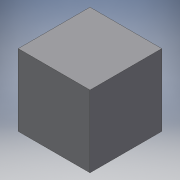
# Autodesk Inventor part: Y screw nut
Saved by Autodesk Inventor 2019 (Build 230136000, 136)
## iProperties
Created: 2018-10-07
Part Number: Y screw nut
Material: Generic
Document SubType Name: Modeling
Designer: LillaHunden
Density: 1 g/cm^3
Appearance: Default
Author: LillaHunden
Autodesk Inventor part; units mm, degrees
ref_plane "YZ Plane" through (0, 0, 0) normal (1, 0, 0) x (0, 1, 0)
ref_plane "XZ Plane" through (0, 0, 0) normal (0, 1, 0) x (-1, 0, 0)
ref_plane "XY Plane" through (0, 0, 0) normal (0, 0, 1) x (1, 0, 0)
sketch "Sketch1" plane through (0, 0, 0) normal (0, 0, 1) x (1, 0, 0)
  line L0 (11, -11) -> (-11, -11)
  line L1 (-11, -11) -> (-11, 11)
  line L2 (-11, 11) -> (11, 11)
  line L3 (11, 11) -> (11, -11)
  circle A0 centre (0, 0) radius 11 construction
  point P0 (0, 0)
  dimension "d0" = 11
  dimension "d2" = 11
  dimension "d3" = 22
  dimension "d4" = 22
  constraints: 8 end point, 2 parallel, 1 horizontal, 1 perpendicular
  measures "d0" distance from line of L0 A0.centre
  measures "d2" distance from line of L3 point (0, 0)
  measures "d3" distance between parallel lines of L3 L1
  measures "d4" distance between parallel lines of L2 L0
extrude "Extrusion1" add sketch "Sketch1" along normal blind 22
sketch "Sketch2" plane through (0, 0, 0) normal (0, 0, -1) x (-1, 0, 0)
  spline S0 degree 3 poles (1.2645, -7.9999) (1.2645, -8.2392) (1.1946, -8.4773) (1.0679, -8.6772) (0.8465, -9.0263) (0.4373, -9.2564) (0.0241, -9.2643) (-0.3891, -9.2722) (-0.8065, -9.058) (-1.0412, -8.7176) (-1.2758, -8.3771) (-1.3274, -7.9108) (-1.1728, -7.5274) (-1.0183, -7.1439) (-0.6567, -6.8433) (-0.2523, -6.7609) (0.1521, -6.6786) (0.6001, -6.8118) (0.8941, -7.1059) knots -5.497425 -5.497425 -5.497425 -5.497425 -4.932647 -4.932647 -4.932647 -3.946117 -3.946117 -3.946117 -2.959588 -2.959588 -2.959588 -1.973059 -1.973059 -1.973059 -0.986529 -0.986529 -0.986529 0 0 0 0 construction
  arc A0 (0.8941, -7.1059) -> (0.8941, -7.1059) centre (0, -8) ccw construction
  spline S1 degree 3 poles (-6.7355, 0.0001) (-6.7355, -0.2392) (-6.8054, -0.4773) (-6.9321, -0.6772) (-7.1535, -1.0263) (-7.5627, -1.2564) (-7.9759, -1.2643) (-8.3891, -1.2722) (-8.8065, -1.058) (-9.0412, -0.7176) (-9.2758, -0.3771) (-9.3274, 0.0892) (-9.1728, 0.4726) (-9.0183, 0.8561) (-8.6567, 1.1567) (-8.2523, 1.2391) (-7.8479, 1.3214) (-7.3999, 1.1882) (-7.1059, 0.8941) knots -5.497425 -5.497425 -5.497425 -5.497425 -4.932647 -4.932647 -4.932647 -3.946117 -3.946117 -3.946117 -2.959588 -2.959588 -2.959588 -1.973059 -1.973059 -1.973059 -0.986529 -0.986529 -0.986529 0 0 0 0 construction
  arc A1 (-7.1059, 0.8941) -> (-7.1059, 0.8941) centre (-8, 0) ccw construction
  spline S2 degree 3 poles (9.2645, 0.0001) (9.2645, -0.2392) (9.1946, -0.4773) (9.0679, -0.6772) (8.8465, -1.0263) (8.4373, -1.2564) (8.0241, -1.2643) (7.6109, -1.2722) (7.1935, -1.058) (6.9588, -0.7176) (6.7242, -0.3771) (6.6726, 0.0892) (6.8272, 0.4726) (6.9817, 0.8561) (7.3433, 1.1567) (7.7477, 1.2391) (8.1521, 1.3214) (8.6001, 1.1882) (8.8941, 0.8941) knots -5.497425 -5.497425 -5.497425 -5.497425 -4.932647 -4.932647 -4.932647 -3.946117 -3.946117 -3.946117 -2.959588 -2.959588 -2.959588 -1.973059 -1.973059 -1.973059 -0.986529 -0.986529 -0.986529 0 0 0 0 construction
  arc A2 (9.2645, 0) -> (8.8941, 0.8941) centre (8, 0) ccw construction
  spline S3 degree 3 poles (1.2645, 8.0001) (1.2645, 7.7608) (1.1946, 7.5227) (1.0679, 7.3228) (0.8465, 6.9737) (0.4373, 6.7436) (0.0241, 6.7357) (-0.3891, 6.7278) (-0.8065, 6.942) (-1.0412, 7.2824) (-1.2758, 7.6229) (-1.3274, 8.0892) (-1.1728, 8.4726) (-1.0183, 8.8561) (-0.6567, 9.1567) (-0.2523, 9.2391) (0.1521, 9.3214) (0.6001, 9.1882) (0.8941, 8.8941) knots -5.497425 -5.497425 -5.497425 -5.497425 -4.932647 -4.932647 -4.932647 -3.946117 -3.946117 -3.946117 -2.959588 -2.959588 -2.959588 -1.973059 -1.973059 -1.973059 -0.986529 -0.986529 -0.986529 0 0 0 0 construction
  arc A3 (1.2645, 8) -> (1.2645, 8) centre (0, 8) ccw construction
  point P0 (0, 0)
  constraints: 4 coincident
hole "Hole1" at (0, -8, 0) at (8, 0, 0) at (-8, 0, 0) at (0, 8, 0) direction (0, 0, 1) diameter 2.459 depth 12.5 tip angle 118
sketch "Sketch3" plane through (0, 0, 22) normal (0, 0, 1) x (1, 0, 0)
  circle A0 centre (0, 0) radius 2.5 construction
  circle A1 centre (0, 0) radius 4.25
  point P0 (0, 0)
  dimension "d14" = 8.5
  constraints: 1 centre point, 1 coincident
  measures "d14" diameter of A1
extrude "Extrusion2" cut sketch "Sketch3" against normal through all
sketch "Sketch4" plane through (-11, -11, 0) normal (0, -1, 0) x (1, 0, 0)
  line L0 (18.5, 18.5) -> (3.5, 18.5) construction
  line L1 (3.5, 18.5) -> (3.5, 3.5) construction
  line L2 (3.5, 3.5) -> (18.5, 3.5) construction
  line L3 (18.5, 3.5) -> (18.5, 18.5) construction
  line L4 (18.5, 18.5) -> (3.5, 3.5) construction
  line L5 (3.5, 18.5) -> (18.5, 3.5) construction
  line L6 (22, 0) -> (22, 22) construction
  line L7 (0, 22) -> (22, 22) construction
  point P0 (11, 0)
  point P1 (11, 11)
  point P2 (18.5, 11)
  point P3 (22, 11)
  point P4 (11, 18.5)
  point P5 (11, 22)
  dimension "d17" = 15
  dimension "d18" = 15
  constraints: 12 end point, 6 midpoint, 4 coincident, 2 parallel, 1 horizontal, 1 horizontal alignment, 1 perpendicular, 1 vertical alignment
  measures "d17" distance of L2.end L1.end
  measures "d18" distance of L1.end L0.end
hole "Hole2" at (7.5, -11, 18.5) at (7.5, -11, 3.5) at (-7.5, -11, 3.5) at (-7.5, -11, 18.5) direction (0, 1, 0) diameter 2.459 depth 12 tip angle 118 thread size "M3x0.5" class "6H" standard "ISO Metric profile"
sketch "Sketch5" plane through (0, 0, 22) normal (0, 0, 1) x (1, 0, 0)
  circle A0 centre (0, 8) radius 1.2295 projected
  circle A1 centre (-8, 0) radius 1.2295 projected
  circle A2 centre (0, -8) radius 1.2295 projected
  circle A3 centre (8, 0) radius 1.2295 projected
  point P0 (0, 0)
extrude "Extrusion3" cut sketch "Sketch5" against normal through all
sketch "Sketch6" plane through (0, 0, 22) normal (0, 0, 1) x (1, 0, 0)
  circle A0 centre (-8, 0) radius 1.2295 construction
  circle A1 centre (0, 8) radius 1.2295 construction
  circle A2 centre (8, 0) radius 1.2295 construction
  circle A3 centre (0, -8) radius 1.2295 construction
  circle A4 centre (-8, 0) radius 2.7295 construction
  circle A5 centre (0, -8) radius 2.7295 construction
  circle A6 centre (8, 0) radius 2.7295 construction
  circle A7 centre (0, 8) radius 2.7295 construction
  circle A8 centre (-8, 0) radius 2.5
  circle A9 centre (0, -8) radius 2.5
  circle A10 centre (8, 0) radius 2.5
  circle A11 centre (0, 8) radius 2.5
  point P0 (0, 0)
  dimension "d28" = 1.5
  dimension "d31" = 360
  dimension "d35" = 5
  dimension "d38" = 360
  constraints: 8 centre point, 1 coincident, 18 other
  measures "d28" radial gap between concentric circles of A0 A4
  measures "d35" diameter of A8
extrude "Extrusion4" cut sketch "Sketch6" against normal blind 10
equation "\"d3\" = 2 * d2"
equation "\"d4\" = 2 * d0"
body "Solid1"
